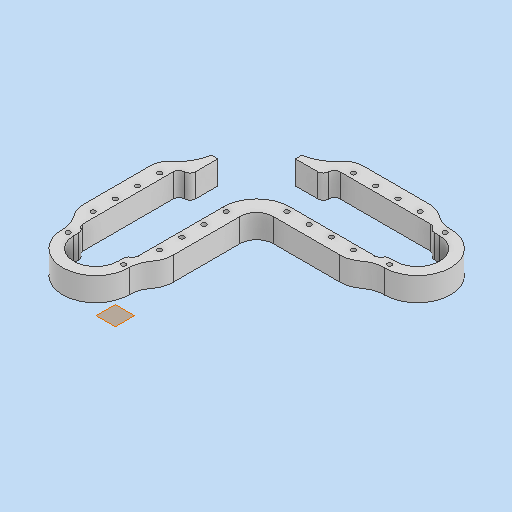
# Autodesk Inventor part: Gearbox Cover Large
Saved by Autodesk Inventor 2024 (Build 280153000, 153)
## iProperties
Created: 2023-09-21
Part Number: Gearbox Cover Large
Material: Generic
Document SubType Name: Modeling
Designer: lando
Density: 1 g/cm^3
Appearance: Default
Author: lando
Autodesk Inventor part; units mm, degrees
ref_plane "YZ Plane" through (0, 0, 0) normal (1, 0, 0) x (0, 1, 0)
ref_plane "XZ Plane" through (0, 0, 0) normal (0, 1, 0) x (-1, 0, 0)
ref_plane "XY Plane" through (0, 0, 0) normal (0, 0, 1) x (1, 0, 0)
ref_plane "Work Plane1" through (153.3626, 3.175, 315.1376) normal (0, 1, 0) x (1, 0, 0)
sketch "Sketch2" plane through (153.3626, 3.175, 315.1376) normal (0, 1, 0) x (1, 0, 0)
  circle A0 centre (-50.8, 212.575) radius 6.35 projected
  line L0 (-50.8, 212.575) -> (-50.8, 187.175)
  line L1 (-50.8, 187.175) -> (-102.9735, 187.175)
  circle A1 centre (-88.9, 139.7) radius 2.65 projected
  circle A2 centre (-88.9, 114.3) radius 2.65 projected
  line L2 (-101.6, 142.5126) -> (-101.6, 66.675) projected
  line L3 (-50.8, 212.575) -> (-25.4, 212.575)
  line L4 (-25.4, 212.575) -> (-25.4, 238.8185)
  line L5 (-101.6, 142.5126) -> (-101.6, 66.675)
  arc A3 (-88.9, 28.575) -> (-12.7, 28.575) centre (-50.8, 28.575) ccw projected
  circle A4 centre (-50.8, 28.575) radius 38.1
  line L6 (-101.6, 66.675) -> (-82.55, 66.675)
  line L7 (-82.55, 45.5611) -> (-82.55, 142.5126)
  arc A5 (-76.2, 28.575) -> (-25.4, 28.575) centre (-50.8, 28.575) ccw
  line L8 (-82.55, 66.675) -> (-76.2, 66.675)
  line L9 (-76.2, 34.5626) -> (-76.2, 28.575)
  line L10 (-101.6, 142.5126) -> (-82.55, 142.5126)
  line L11 (-82.55, 40.9126) -> (-82.55, 40.9126)
  arc A6 (-76.2, 34.5626) -> (-79.375, 40.0618) centre (-82.55, 34.5626) ccw
  arc A7 (-82.55, 45.5611) -> (-79.375, 40.0618) centre (-76.2, 45.5611) ccw
  line L12 (-82.55, 142.5126) -> (-82.55, 148.8626)
  line L13 (-76.2, 155.2126) -> (-76.2, 155.2126)
  line L14 (-69.85, 161.5626) -> (-69.85, 187.175)
  arc A8 (-76.2, 155.2126) -> (-69.85, 161.5626) centre (-76.2, 161.5626) ccw
  arc A9 (-76.2, 155.2126) -> (-82.55, 148.8626) centre (-76.2, 148.8626) ccw
  line L15 (-19.05, 45.5611) -> (-19.05, 142.5126)
  line L16 (-25.4, 34.5626) -> (-25.4, 28.575)
  arc A10 (-22.225, 40.0618) -> (-25.4, 34.5626) centre (-19.05, 34.5626) ccw
  arc A11 (-22.225, 40.0618) -> (-19.05, 45.5611) centre (-25.4, 45.5611) ccw
  arc A12 (19.05, 161.775) -> (0, 142.725) centre (19.05, 142.725) ccw projected
  circle A13 centre (19.05, 142.725) radius 19.05
  circle A14 centre (19.05, 142.725) radius 38.1006
  line L17 (-50.8, 212.575) -> (-25.4, 212.575)
  line L18 (-25.4, 212.575) -> (-25.4, 264.7485)
  circle A15 centre (22.075, 250.675) radius 2.65
  circle A16 centre (47.475, 250.675) radius 2.65
  line L19 (19.2624, 263.375) -> (95.1, 263.375)
  line L20 (-50.8, 212.575) -> (-50.8, 187.175)
  line L21 (19.2624, 263.375) -> (95.1, 263.375)
  arc A17 (133.2, 174.475) -> (133.2, 250.675) centre (133.2, 212.575) ccw
  circle A18 centre (133.2, 212.575) radius 38.1
  line L22 (95.1, 263.375) -> (95.1, 244.325)
  line L23 (116.2139, 244.325) -> (19.2624, 244.325)
  arc A19 (133.2, 187.175) -> (133.2, 237.975) centre (133.2, 212.575) ccw
  line L24 (95.1, 244.325) -> (95.1, 237.975)
  line L25 (127.2124, 237.975) -> (133.2, 237.975)
  line L26 (120.8624, 244.325) -> (120.8624, 244.325)
  arc A20 (121.7132, 241.15) -> (127.2124, 237.975) centre (127.2124, 244.325) ccw
  arc A21 (121.7132, 241.15) -> (116.2139, 244.325) centre (116.2139, 237.975) ccw
  line L27 (19.2624, 244.325) -> (12.9124, 244.325)
  line L28 (6.5624, 237.975) -> (6.5624, 237.975)
  line L29 (0.2124, 231.625) -> (-25.4, 231.625)
  arc A22 (0.2124, 231.625) -> (6.5624, 237.975) centre (0.2124, 237.975) ccw
  arc A23 (12.9124, 244.325) -> (6.5624, 237.975) centre (12.9124, 237.975) ccw
  line L30 (116.2139, 180.825) -> (19.2624, 180.825)
  arc A24 (127.2124, 187.175) -> (121.7132, 184) centre (127.2124, 180.825) ccw
  arc A25 (116.2139, 180.825) -> (121.7132, 184) centre (116.2139, 187.175) ccw
  line L31 (127.2124, 187.175) -> (133.2, 187.175)
  arc A26 (-34.6191, 237.975) -> (4.5675, 256.4477) centre (-34.6191, 288.775) ccw projected
  arc A27 (-25.4, 238.8185) -> (4.5675, 256.4477) centre (-34.6191, 288.775) ccw
  arc A28 (19.2624, 263.375) -> (4.5675, 256.4477) centre (19.2624, 244.325) ccw projected
  arc A29 (19.2624, 263.375) -> (4.5675, 256.4477) centre (19.2624, 244.325) ccw
  line L32 (0, 66.675) -> (0, 142.725) projected
  line L33 (0, 142.725) -> (0, 25.7278)
  arc A30 (-94.6727, 157.2075) -> (-101.6, 142.5126) centre (-82.55, 142.5126) ccw projected
  arc A31 (-94.6727, 157.2075) -> (-101.6, 142.5126) centre (-82.55, 142.5126) ccw
  arc A32 (-94.6727, 157.2075) -> (-76.2, 196.3941) centre (-127, 196.3941) ccw projected
  arc A33 (-94.6727, 157.2075) -> (-76.2, 196.3941) centre (-127, 196.3941) ccw
  line L34 (19.05, 161.775) -> (95.1, 161.775)
  line L35 (-101.6, 66.675) -> (-101.6, 47.625) construction
  line L36 (-101.6, 47.625) -> (-88.9, 47.625) construction
  line L37 (-88.9, 47.625) -> (-88.9, 28.575) construction
  spline S0 degree 3 poles (-101.6, 66.675) (-101.6, 47.625) (-88.9, 47.625) (-88.9, 28.575) knots 1 1 1 1 2 2 2 2
  line L38 (-50.8, 28.575) -> (-50.8, 60.9646)
  spline S1 degree 3 poles (0, 66.675) (0, 47.625) (-12.7, 47.625) (-12.7, 28.575) knots 1 1 1 1 2 2 2 2
  line L39 (0, 66.675) -> (0, 47.625) construction
  line L40 (0, 47.625) -> (-12.7, 47.625) construction
  line L41 (-12.7, 47.625) -> (-12.7, 28.575) construction
  spline S2 degree 3 poles (95.1, 263.375) (114.15, 263.375) (114.15, 250.675) (133.2, 250.675) knots 1 1 1 1 2 2 2 2
  line L42 (95.1, 263.375) -> (114.15, 263.375) construction
  line L43 (114.15, 263.375) -> (114.15, 250.675) construction
  line L44 (114.15, 250.675) -> (133.2, 250.675) construction
  spline S3 degree 3 poles (95.1, 161.775) (114.15, 161.775) (114.15, 174.475) (133.2, 174.475) knots 1 1 1 1 2 2 2 2
  line L45 (95.1, 161.775) -> (114.15, 161.775) construction
  line L46 (114.15, 161.775) -> (114.15, 174.475) construction
  line L47 (114.15, 174.475) -> (133.2, 174.475) construction
  circle A34 centre (-88.9, 88.9) radius 2.65 projected
  circle A35 centre (-88.9, 88.9) radius 2.65
  circle A36 centre (-88.9, 63.5) radius 2.65 projected
  circle A37 centre (-88.9, 63.5) radius 2.65
  circle A38 centre (-82.55, 28.575) radius 2.65 projected
  circle A39 centre (-82.55, 28.575) radius 2.65
  circle A40 centre (-19.05, 28.575) radius 2.65 projected
  circle A41 centre (-19.05, 28.575) radius 2.65
  circle A42 centre (-12.7, 63.5) radius 2.65 projected
  circle A43 centre (-12.7, 63.5) radius 2.65
  circle A44 centre (-12.7, 88.9) radius 2.65 projected
  circle A45 centre (-12.7, 88.9) radius 2.65
  circle A46 centre (-12.7, 114.3) radius 2.65 projected
  circle A47 centre (-12.7, 114.3) radius 2.65
  circle A48 centre (-12.7, 139.7) radius 2.65 projected
  circle A49 centre (-12.7, 139.7) radius 2.65
  circle A50 centre (22.075, 174.475) radius 2.65 projected
  circle A51 centre (22.075, 174.475) radius 2.65
  circle A52 centre (47.475, 174.475) radius 2.65 projected
  circle A53 centre (47.475, 174.475) radius 2.65
  circle A54 centre (72.875, 174.475) radius 2.65 projected
  circle A55 centre (72.875, 174.475) radius 2.65
  circle A56 centre (98.275, 174.475) radius 2.65 projected
  circle A57 centre (98.275, 174.475) radius 2.65
  circle A58 centre (133.2, 180.825) radius 2.65 projected
  circle A59 centre (133.2, 180.825) radius 2.65
  circle A60 centre (133.2, 244.325) radius 2.65 projected
  circle A61 centre (133.2, 244.325) radius 2.65
  circle A62 centre (98.275, 250.675) radius 2.65 projected
  circle A63 centre (98.275, 250.675) radius 2.65
  circle A64 centre (72.875, 250.675) radius 2.65
  point P0 (-153.3626, 315.1376)
  point P1 (-82.55, 155.2126)
  point P2 (-69.85, 155.2126)
  point P3 (6.5624, 244.325)
  point P4 (6.5624, 231.625)
  point P5 (-77.0435, 187.175)
  point P6 (-88.9, 28.575)
  point P7 (-12.7, 28.575)
  point P8 (133.2, 174.475)
  point P9 (133.2, 250.675)
  point P10 (-25.4, 238.8185)
  point P11 (6.5624, 237.975)
  point P12 (19.2624, 244.325)
  dimension "d40" = 25.4
  dimension "d43" = 19.05
  dimension "d46" = 12.7
  dimension "d47" = 76.2
  dimension "d48" = 101.6
  dimension "d49" = 6.35
  dimension "d50" = 12.7
  dimension "d51" = 12.7
  dimension "d52" = 6.35
  dimension "d53" = 19.05
  dimension "d54" = 19.05
  constraints: 68 end point, 41 centre point, 41 point on circle, 19 coincident, 15 point on line, 9 perpendicular, 9 tangent, 5 vertical, 4 horizontal, 4 symmetric about line, 2 concentric, 2 equal radius, 1 parallel, 12 other
  measures "d40" distance of L0.start L0.end
  measures "d43" distance of L6.end L2.end
  measures "d46" radial gap between concentric circles of A3 A5
  measures "d47" diameter of A4
  measures "d48" distance of L11.start L7.end
  measures "d49" radius of A6
  measures "d50" distance of L10.end point (-82.55, 155.213)
  measures "d51" distance of point (-82.55, 155.213) point (-69.85, 155.213)
  measures "d52" radius of A8
  measures "d53" distance of L35.start L35.end
  measures "d54" distance of L37.end L36.end
extrude "Extrusion2" add sketch "Sketch2" along normal blind 26.924 contours L4 A26 A28 L19 L22 L23 L27 A23 A22 L29 | L14 A8 A9 L12 L10 A30 A32 L1 | L10 L7 L6 L2 | S2 A18 L23 L22 | L6 L7 A4 S0 | A17 A18 L30 A25 A24 L31 A19 L25 A20 A21 L23 | A4 L7 A7 A6 L9 A5 L16 A10 A11 L15 A3 | A4 L15 A14 L32 S1 | A18 S3 L34 A14 L30 | A14 L34 A12 L32
body "Solid1"
